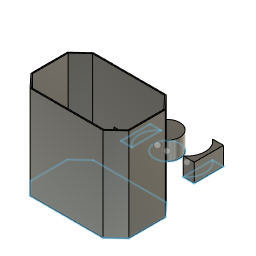
robot model 3D v5 (Autodesk Fusion 360 design; units mm, degrees)
Autodesk Fusion 360 part; units mm, degrees
sketch "Esquisse1" plane through (0, 0, 0) normal (0, 0, 1) x (1, 0, 0)
  line L0 (-97.4947, 52.0667) -> (102.5053, 52.0667)
  line L1 (102.5053, 52.0667) -> (136.5995, 15.4937)
  line L2 (136.5995, 15.4937) -> (136.5995, -84.5063)
  line L3 (136.5995, -84.5063) -> (100.0264, -118.6005)
  line L4 (100.0264, -118.6005) -> (-99.9736, -118.6005)
  line L5 (-99.9736, -118.6005) -> (-134.0677, -82.0275)
  line L6 (-134.0677, -82.0275) -> (-134.0677, 17.9725)
  line L7 (-134.0677, 17.9725) -> (-97.4947, 52.0667)
  circle A0 centre (-18.2616, 175) radius 35
  line L8 (95.6977, 135.6449) -> (65.6977, 135.6449)
  line L9 (65.6977, 135.6449) -> (65.6977, 215.6449)
  line L10 (65.6977, 215.6449) -> (95.6977, 215.6449)
  line L11 (95.6977, 215.6449) -> (95.6977, 135.6449)
  line L12 (-105.2122, 215.6449) -> (-75.2122, 215.6449)
  line L13 (-105.2122, 135.6449) -> (-105.2122, 215.6449)
  line L14 (-75.2122, 215.6449) -> (-75.2122, 135.6449)
  line L15 (-75.2122, 135.6449) -> (-105.2122, 135.6449)
  arc A1 (65.6977, 135.6449) -> (65.6977, 215.6449) centre (35.6977, 175.6449) ccw
  arc A2 (-75.2122, 215.6449) -> (-75.2122, 135.6449) centre (-45.2122, 175.6449) ccw
  dimension "d1" = 100
  dimension "d4" = 200
  dimension "d5" = 50
  dimension "d6" = 170.6672
  dimension "d7" = 270.6672
  dimension "d44" = 70
  dimension "d48" = 30
  dimension "d49" = 80
  dimension "d52" = 30
  dimension "d53" = 80
  dimension "d57" = 60
  dimension "d58" = 60
  constraint perpendicular L5 L7
  constraint equal L3 L5
  constraint equal L1 L7
  constraint equal L1 L3
  constraint equal L2 L6
  constraint equal L0 L4
  constraint horizontal L8
  constraint vertical L9
  constraint horizontal L10
  constraint vertical L11
  constraint horizontal L15
  constraint vertical L13
  constraint horizontal L12
  constraint vertical L14
  constraint collinear L10 L12
  measures "d1" distance of L1.end L2.end
  measures "d4" distance of L0.start L0.end
  measures "d5" distance of L0.end L1.end
  measures "d6" distance of L0 L4
  measures "d7" distance of L2 L6
  measures "d44" diameter of A0
  measures "d48" distance of L8.start L8.end
  measures "d49" distance of L8.end L9.end
  measures "d52" distance of L14.end L13.start
  measures "d53" distance of L13.start L12.start
  measures "d57" distance of L13 A2.centre
  measures "d58" distance of L11 A1.centre
extrude "Extrusion1" add sketch "Esquisse1" along normal blind 5 contours L0 L1 L2 L3 L4 L5 L6 L7 makes body 1
sketch "Esquisse4" plane through (0, 0, 5) normal (0, 0, 1) x (-1, 0, 0)
  line L0 (134.0677, -17.9725) -> (134.0677, 82.0275)
  line L1 (134.0677, 82.0275) -> (99.9736, 118.6005)
  line L2 (99.9736, 118.6005) -> (-100.0264, 118.6005)
  line L3 (-100.0264, 118.6005) -> (-136.5995, 84.5063)
  line L4 (-136.5995, 84.5063) -> (-136.5995, -15.4937)
  line L5 (-136.5995, -15.4937) -> (-102.5053, -52.0667)
  line L6 (-102.5053, -52.0667) -> (97.4947, -52.0667)
  line L7 (97.4947, -52.0667) -> (134.0677, -17.9725)
  line L8 (96.3133, -49.0667) -> (-101.2006, -49.0667)
  line L9 (97.4947, -52.0667) -> (-102.5053, -52.0667)
  line L10 (-101.2006, -49.0667) -> (-133.5995, -14.3122)
  line L11 (-133.5995, -14.3122) -> (-133.5995, 83.2016)
  line L12 (-102.5053, -52.0667) -> (-136.5995, -15.4937)
  line L13 (-136.5995, -15.4937) -> (-136.5995, 84.5063)
  line L14 (-133.5995, 83.2016) -> (-98.845, 115.6005)
  line L15 (-98.845, 115.6005) -> (98.6688, 115.6005)
  line L16 (98.6688, 115.6005) -> (131.0677, 80.846)
  line L17 (131.0677, 80.846) -> (131.0677, -16.6678)
  line L18 (131.0677, -16.6678) -> (96.3133, -49.0667)
  line L19 (-136.5995, 84.5063) -> (-100.0264, 118.6005)
  line L20 (-100.0264, 118.6005) -> (99.9736, 118.6005)
  line L21 (99.9736, 118.6005) -> (134.0677, 82.0275)
  line L22 (134.0677, 82.0275) -> (134.0677, -17.9725)
  line L23 (134.0677, -17.9725) -> (97.4947, -52.0667)
  line L24 (43.7344, 105.6005) -> (-46.2656, 105.6005)
  line L25 (-46.2656, 105.6005) -> (-46.2656, 35.6005)
  line L26 (-46.2656, 35.6005) -> (43.7344, 35.6005)
  line L27 (43.7344, 35.6005) -> (43.7344, 105.6005)
  line L28 (47.7344, 35) -> (47.7344, 105)
  line L29 (47.7344, 105) -> (47.7344, 109.6005)
  line L30 (47.7344, 109.6005) -> (-50.2656, 109.6005)
  line L31 (-50.2656, 109.6005) -> (-50.2656, 31.6005)
  line L32 (-50.2656, 31.6005) -> (47.7344, 31.6005)
  line L33 (47.7344, 31.6005) -> (47.7344, 35)
  dimension "d10" = 3
  dimension "d11" = 3
  dimension "d12" = 3
  dimension "d14" = 3
  dimension "d16" = 3
  dimension "d18" = 3
  dimension "d19" = 3
  dimension "d21" = 3
  dimension "d24" = 70
  dimension "d25" = 90
  dimension "d26" = 10
  dimension "d27" = 4
  dimension "d28" = 4
  dimension "d29" = 4
  dimension "d30" = 4
  dimension "d35" = 83.3333
  dimension "d36" = 83.3339
  constraint parallel L6 L8
  constraint parallel L5 L10
  constraint perpendicular L8 L11
  constraint parallel L11 L17
  constraint horizontal L24
  constraint vertical L25
  constraint horizontal L26
  constraint vertical L27
  constraint parallel L27 L28
  constraint parallel L28 L29
  constraint perpendicular L29 L30
  constraint perpendicular L30 L31
  constraint perpendicular L31 L32
  constraint perpendicular L32 L33
  measures "d10" distance of L8 L9
  measures "d11" distance of L10 L12
  measures "d12" distance of L11 L13
  measures "d14" distance of L14 L19
  measures "d16" distance of L15 L20
  measures "d18" distance of L16 L21
  measures "d19" distance of L17 L22
  measures "d21" distance of L18 L23
  measures "d24" distance of L24.end L25.end
  measures "d25" distance of L25.end L26.end
  measures "d26" distance of L15 L24
  measures "d27" distance of L27 L28
  measures "d28" distance of L25 L31
  measures "d29" distance of L26 L32
  measures "d30" distance of L24 L30
  measures "d35" distance of L17 L28
  measures "d36" distance of L11 L31
extrude "Extrusion2" add sketch "Esquisse4" along normal blind 250 contours L0 L1 L2 L3 L4 L5 L6 L7 L9 L12 L13 L19 L20 L21 L22 L23 bodies 1
extrude "Extrusion3" add sketch "Esquisse4" along normal blind 5 contours L28 L29 L30 L31 L32 L33 bodies 1
extrude "Extrusion4" add 1 faces at (16.2656, -108.2672, 10) along direction (0, 0, 1) blind 5 on bodies 1 bodies 1
sketch "Esquisse5" plane through (0, 52.0667, 0) normal (0, 1, 0) x (-1, 0, 0)
  line L0 (-102.5053, 0) -> (97.4947, 0)
  line L1 (97.4947, 0) -> (97.4947, 255)
  line L2 (97.4947, 255) -> (-102.5053, 255)
  line L3 (-102.5053, 255) -> (-102.5053, 0)
  line L4 (-42.5053, 10) -> (37.4947, 10)
  line L5 (37.4947, 10) -> (37.4947, 110)
  line L6 (37.4947, 110) -> (-42.5053, 110)
  line L7 (-42.5053, 110) -> (-42.5053, 10)
  line L8 (97.4947, 0) -> (-102.5053, 0)
  dimension "d37" = 10
  dimension "d38" = 80
  dimension "d39" = 100
  dimension "d40" = 60
  dimension "d41" = 60
  constraint horizontal L4
  constraint vertical L5
  constraint horizontal L6
  constraint vertical L7
  measures "d37" distance of L4 L8
  measures "d38" distance of L4.start L4.end
  measures "d39" distance of L4.start L6.end
  measures "d40" distance of L3 L7
  measures "d41" distance of L1 L5
extrude "Extrusion5" cut sketch "Esquisse5" against normal blind 20 contours L4 L5 L6 L7 bodies 1
extrude "Extrusion6" add sketch "Esquisse1" along normal blind 50 separate body contours A0 makes body 2
extrude "Extrusion7" add sketch "Esquisse1" along normal blind 50 separate body contours L8 L10 L11 A1 | L12 L13 L15 A2 makes body 3 at (-94.5212, 183.9284, 33.3333) makes body 4 at (69.3607, 212.6152, 33.3333)
